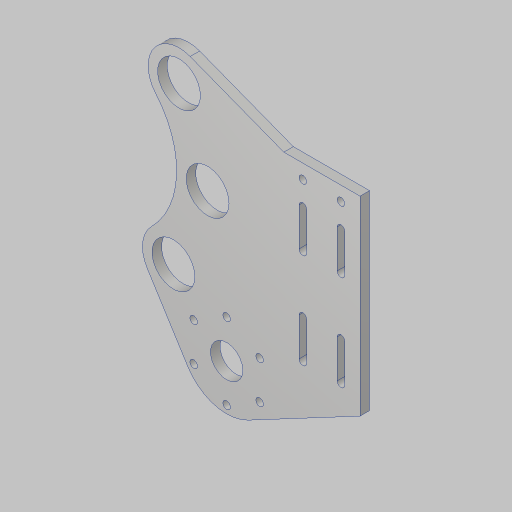
# Autodesk Inventor part: CL7-GB-002
Saved by Autodesk Inventor 2023.5 (Build 275446000, 446)
## iProperties
Created: 2025-03-18
Part Number: CL7-GB-002
Material: Aluminum 6061
Document SubType Name: Modeling
Designer: slick
Density: 2.7 g/cm^3
Appearance: Aluminum - Flat
Author: slick
Autodesk Inventor part; units mm, degrees
ref_plane "YZ Plane" through (0, 0, 0) normal (1, 0, 0) x (0, 1, 0)
ref_plane "XZ Plane" through (0, 0, 0) normal (0, 1, 0) x (-1, 0, 0)
ref_plane "XY Plane" through (0, 0, 0) normal (0, 0, 1) x (1, 0, 0)
sketch "Sketch1" plane through (0, 0, 0) normal (0, 0, 1) x (1, 0, 0)
  line L0 (0, 0) -> (-50.8, 0) construction
  line L1 (-50.8, 0) -> (-50.8, 381) construction
  line L2 (-50.8, 381) -> (0, 381) construction
  line L3 (0, 381) -> (0, 0) construction
  circle A0 centre (-50.8, 431.8) radius 11.1125 construction
  line L4 (-50.8, 353.7099) -> (-298.4703, 0) construction
  line L5 (-298.4703, 0) -> (-267.4626, 0) construction
  line L6 (-267.4626, 0) -> (-50.8, 309.4263) construction
  dimension "d0" = 50.8
  dimension "d1" = 381
  dimension "d2" = 22.225
  dimension "d3" = 431.8
  dimension "d4" = 50.8
  dimension "d5" = 431.8
  dimension "d6" = 25.4
  dimension "d7" = 35
  constraints: 14 end point, 3 parallel, 2 horizontal, 2 point on line, 1 centre point, 1 collinear, 1 perpendicular
  measures "d0" distance of L1.end L2.end
  measures "d1" distance of L0.end L1.end
  measures "d2" diameter of A0
  measures "d3" distance from line of L0 A0.centre
  measures "d4" distance from line of L3 A0.centre
  measures "d5" distance of L4.start L4.end
  measures "d6" distance between parallel lines of L6 L4
  measures "d7" angle of L1 L4
sketch "Sketch2" plane through (0, 0, 0) normal (0, 0, 1) x (1, 0, 0)
  line L0 (-267.4626, 0) -> (-50.8, 309.4263) construction
  line L1 (-50.8, 353.7099) -> (-298.4703, 0) construction
  line L2 (-50.8, 0) -> (-50.8, 381) construction
  line L3 (0, 381) -> (0, 0) construction
  line L4 (-50.8, 381) -> (0, 381) construction
  circle A0 centre (-50.8, 431.8) radius 11.1125 construction
  line L5 (0, 0) -> (-50.8, 0) construction
  line L6 (-298.4703, 0) -> (-267.4626, 0) construction
  circle A1 centre (-88.9, 38.1) radius 30.48 construction
  circle A2 centre (-88.9, 38.1) radius 6.35 construction
  circle A3 centre (-124.3919, 76.2) radius 45.72 construction
  circle A4 centre (-124.3919, 76.2) radius 11.43 construction
  circle A5 centre (-101.6, 129.9906) radius 46.99 construction
  circle A6 centre (-101.6, 129.9906) radius 12.7 construction
  circle A7 centre (-120.65, 182.5232) radius 43.18 construction
  circle A8 centre (-124.3919, 76.2) radius 14.2875
  circle A9 centre (-101.6, 129.9906) radius 14.2875
  circle A10 centre (-120.65, 182.5232) radius 14.2875
  circle A11 centre (-50.8, 431.8) radius 54.5719 construction
  line L7 (-50.8, 177.8) -> (0, 177.8)
  circle A12 centre (-120.65, 182.5232) radius 20.6375 construction
  circle A13 centre (-101.6, 129.9906) radius 20.6375 construction
  circle A14 centre (-124.3919, 76.2) radius 20.6375 construction
  circle A15 centre (-88.9, 38.1) radius 25.4 construction
  line L8 (-50.8, 177.8) -> (-113.2499, 201.7883)
  line L9 (-141.8793, 65.2411) -> (-114.7275, 21.9145)
  line L10 (-74.6041, 11.1805) -> (0, 50.8)
  line L11 (0, 177.8) -> (0, 50.8)
  arc A16 (-139.0075, 90.7702) -> (-136.2537, 169.0164) centre (-179.7388, 131.3753) ccw
  arc A17 (-113.2499, 201.7883) -> (-136.2537, 169.0164) centre (-120.65, 182.5232) ccw
  arc A18 (-139.0075, 90.7702) -> (-141.8793, 65.2411) centre (-124.3919, 76.2) ccw
  arc A19 (-114.7275, 21.9145) -> (-74.6041, 11.1805) centre (-88.9, 38.1) ccw
  line L12 (-38.1, 152.4) -> (-38.1, 127) construction
  line L13 (-40.6527, 152.4) -> (-40.6527, 127)
  line L14 (-35.5473, 127) -> (-35.5473, 152.4)
  arc A20 (-35.5473, 152.4) -> (-40.6527, 152.4) centre (-38.1, 152.4) ccw
  arc A21 (-40.6527, 127) -> (-35.5473, 127) centre (-38.1, 127) ccw
  line L15 (-12.7, 152.4) -> (-12.7, 127) construction
  line L16 (-15.2527, 152.4) -> (-15.2527, 127)
  line L17 (-10.1473, 127) -> (-10.1473, 152.4)
  arc A22 (-10.1473, 152.4) -> (-15.2527, 152.4) centre (-12.7, 152.4) ccw
  arc A23 (-15.2527, 127) -> (-10.1473, 127) centre (-12.7, 127) ccw
  line L18 (-38.1, 139.7) -> (-12.7, 139.7) construction
  line L19 (-38.1, 88.9) -> (-38.1, 63.5) construction
  line L20 (-40.6527, 88.9) -> (-40.6527, 63.5)
  line L21 (-35.5473, 63.5) -> (-35.5473, 88.9)
  arc A24 (-35.5473, 88.9) -> (-40.6527, 88.9) centre (-38.1, 88.9) ccw
  arc A25 (-40.6527, 63.5) -> (-35.5473, 63.5) centre (-38.1, 63.5) ccw
  line L22 (-12.7, 88.9) -> (-12.7, 63.5) construction
  line L23 (-15.2527, 88.9) -> (-15.2527, 63.5)
  line L24 (-10.1473, 63.5) -> (-10.1473, 88.9)
  arc A26 (-10.1473, 88.9) -> (-15.2527, 88.9) centre (-12.7, 88.9) ccw
  arc A27 (-15.2527, 63.5) -> (-10.1473, 63.5) centre (-12.7, 63.5) ccw
  line L25 (-38.1, 76.2) -> (-12.7, 76.2) construction
  circle A28 centre (-88.9, 38.1) radius 10.795
  point P0 (-88.9, 63.5)
  point P1 (-110.897, 50.8)
  point P2 (-110.897, 25.4)
  point P3 (-88.9, 12.7)
  point P4 (-66.903, 25.4)
  point P5 (-66.903, 50.8)
  point P6 (-25.4, 139.7)
  point P7 (-25.4, 177.8)
  point P8 (-25.4, 76.2)
  point P9 (-38.1, 168.275)
  point P10 (-12.7, 168.275)
  dimension "d25" = 50.8
  dimension "d8" = 60.96
  dimension "d9" = 12.7
  dimension "d10" = 91.44
  dimension "d11" = 38.1
  dimension "d12" = 38.1
  dimension "d13" = 22.86
  dimension "d14" = 93.98
  dimension "d15" = 25.4
  dimension "d16" = 86.36
  dimension "d17" = 76.2
  dimension "d20" = 50.8
  dimension "d21" = 19.05
  dimension "d22" = 28.575
  dimension "d23" = 109.1438
  dimension "d24" = 6.35
  dimension "d28" = 360
  dimension "d30" = 177.8
  dimension "d31" = 50.8
  dimension "d32" = 5.1054
  dimension "d33" = 25.4
  dimension "d34" = 38.1
  dimension "d35" = 25.4
  dimension "d36" = 5.1054
  dimension "d37" = 25.4
  dimension "d38" = 25.4
  dimension "d39" = 63.5
  dimension "d42" = 21.59
  dimension "d50" = 9.525
  constraints: 46 end point, 30 point on circle, 27 centre point, 26 tangent, 14 coincident, 7 midpoint, 6 equal radius, 6 parallel, 6 vertical alignment, 5 horizontal alignment, 3 horizontal, 3 point on line, 2 vertical, 1 collinear, 9 other
  measures "d8" diameter of A1
  measures "d9" diameter of A2
  measures "d10" diameter of A3
  measures "d11" distance from line of L5 A1.centre
  measures "d12" distance from line of L2 A1.centre
  measures "d13" diameter of A4
  measures "d14" diameter of A5
  measures "d15" diameter of A6
  measures "d16" diameter of A7
  measures "d17" distance from line of L5 A3.centre
  measures "d20" distance from line of L2 A5.centre
  measures "d21" horizontal distance of A5.centre A7.centre
  measures "d22" diameter of A8
  measures "d23" diameter of A11
  measures "d24" radial gap between concentric circles of A10 A12
  measures "d30" distance between parallel lines of L5 L7
  measures "d31" distance from line of L5 L10.end
  measures "d32" diameter of A21
  measures "d33" distance of L12.start L12.end
  measures "d34" distance from line of L7 L18.start
  measures "d35" distance of L18.start L18.end
  measures "d36" diameter of A25
  measures "d37" distance of L19.start L19.end
  measures "d38" distance of L25.start L25.end
  measures "d39" distance between parallel lines of L18 L25
  measures "d42" diameter of A28
  measures "d50" distance from line of L7 point (-38.1, 168.275)
extrude "Extrusion1" add sketch "Sketch2" along normal blind 6.35
hole "Hole1" at (-88.9, 63.5, 0) at (-110.897, 50.8, 0) at (-110.897, 25.4, 0) at (-88.9, 12.7, 0) at (-66.903, 25.4, 0) at (-66.903, 50.8, 0) at (-38.1, 168.275, 0) at (-12.7, 168.275, 0) direction (0, 0, 1) diameter 5.1054 end through all clearance for "Flat Head Machine Screw (82)" size "#10" standard "Ansi Unified Screw Threads"
body "Solid1"
